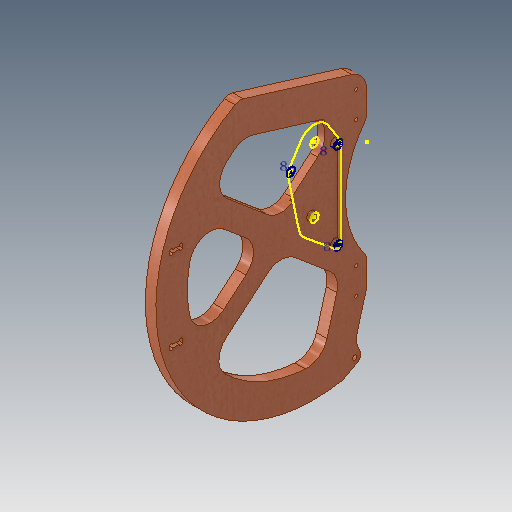
# Autodesk Inventor part: Tplate
Saved by Autodesk Inventor 2019.4 (Build 234330000, 330)
## iProperties
Created: 2019-06-12
Part Number: Tplate
Material: 木材(クルミ)
Document SubType Name: Modeling
Designer: AzLIer
Density: 0.55 g/cm^3
Appearance: クルミ材 - ナチュラル つや出し
Mass: 145.761 g
Surface Area: 731.193 cm^2
Volume: 265.02 cm^3
Author: AzLIer
Autodesk Inventor part; units mm, degrees
(part 1 of 3)
ref_plane "YZ Plane" through (0, 0, 0) normal (1, 0, 0) x (0, 1, 0)
ref_plane "XZ Plane" through (0, 0, 0) normal (0, 1, 0) x (-1, 0, 0)
ref_plane "XY Plane" through (0, 0, 0) normal (0, 0, 1) x (1, 0, 0)
sketch "スケッチ2" plane through (0, 0, 0) normal (1, 0, 0) x (0, 1, 0)
  line L0 (151.996, 0) -> (-248.004, 0)
  line L1 (-248.004, 0) -> (-248.004, 200)
  line L2 (-248.004, 200) -> (151.996, 200)
  line L3 (151.996, 200) -> (151.996, 0)
  point P0 (0, 0)
  dimension "d5" = 400
  dimension "d6" = 200
  constraints: 8 end point, 2 parallel, 1 horizontal, 1 perpendicular, 1 point on line
  measures "d5" distance of L1.end L2.end
  measures "d6" distance of L0.end L1.end
extrude "押し出し2" add sketch "スケッチ2" along normal blind 10
sketch "スケッチ3" plane through (10, 0, 0) normal (1, 0, 0) x (0, 0, -1)
  circle A0 centre (-50, 24.7653) radius 4 projected
  circle A1 centre (-50, -37.0469) radius 4 projected
  circle A2 centre (-72.5, 11.9531) radius 1.6 projected
  circle A3 centre (-27.5, -71.0469) radius 1.6 projected
  circle A4 centre (-27.5, 11.9531) radius 1.6 projected
  line L0 (-62.6183, 32.8757) -> (-75.0237, 13.5752) projected
  arc A5 (-75.0237, 13.5752) -> (-75.4366, 11.3394) centre (-72.5, 11.9531) ccw projected
  line L1 (-75.4366, 11.3394) -> (-64.6828, -40.1155) projected
  arc A6 (-64.6828, -40.1155) -> (-59.5184, -48.64) centre (-50, -37.0469) ccw projected
  line L2 (-59.5184, -48.64) -> (-29.4037, -73.3655) projected
  arc A7 (-29.4037, -73.3655) -> (-24.5, -71.0469) centre (-27.5, -71.0469) ccw projected
  line L3 (-24.5, -71.0469) -> (-24.5, 11.9531) projected
  arc A8 (-24.5, 11.9531) -> (-24.9763, 13.5752) centre (-27.5, 11.9531) ccw projected
  line L4 (-24.9763, 13.5752) -> (-37.3817, 32.8757) projected
  arc A9 (-37.3817, 32.8757) -> (-62.6183, 32.8757) centre (-50, 24.7653) ccw projected
  circle A10 centre (-27.5, -71.0469) radius 4
  circle A11 centre (-72.5, 11.9531) radius 4
  circle A12 centre (-27.5, 11.9531) radius 4
  point P0 (0, 0)
  dimension "d11" = 8
  dimension "d12" = 8
  dimension "d13" = 8
  constraints: 3 centre point, 3 coincident
  measures "d11" diameter of A10
  measures "d12" diameter of A11
  measures "d13" diameter of A12
extrude "押し出し3" cut sketch "スケッチ3" against normal blind 10 contours A0 | A1 | A2 | A3 | A4 | A11 L1 A5 L0 | L0 A5 L1 A11 | A12 L3 A8 L4 | L4 A8 L3 A12 | A10 L2 A7 L3 | L3 A7 L2 A10
extrude "押し出し4" cut sketch "スケッチ3" against normal blind 3 contours A9 L4 A12 L3 A10 L2 A6 L1 A11 L0 | A11 L1 A5 L0 | L4 A8 L3 A12 | L3 A7 L2 A10 picked at (-74.6765, 10.327) picked at (-25.0278, 10.8233) picked at (-25.0278, -69.9171)
sketch "スケッチ4" plane through (0, 0, 0) normal (-1, 0, 0) x (0, 0, 1)
  arc A0 (23.9528, -184.768) -> (125, 92.8569) centre (50, -37.0469) ccw projected
  circle A1 centre (50, -37.0469) radius 150
  point P0 (0, 0)
  constraints: 1 centre point, 1 coincident, 1 concentric
extrude "押し出し5" cut sketch "スケッチ4" against normal through all keep common part
sketch "スケッチ5" plane through (0, 0, 0) normal (-1, 0, 0) x (0, 0, 1)
  line L0 (0, 57.9531) -> (20, 57.9531) projected
  arc A0 (23.9528, -184.768) -> (125, 92.8569) centre (50, -37.0469) ccw projected
  arc A1 (27.4257, -165.0719) -> (23.9528, -184.768) centre (25.6893, -174.92) ccw projected
  arc A2 (27.4257, -165.0719) -> (115, 75.5364) centre (50, -37.0469) ccw projected
  arc A3 (125, 92.8569) -> (115, 75.5364) centre (120, 84.1967) ccw projected
  line L1 (0, 57.9531) -> (117.0753, 93.7594)
  line L2 (0, -120) -> (16.0565, -177.605)
  line L3 (0, 57.9531) -> (0, -120)
  point P0 (0, 0)
  dimension "d57" = 120
  constraints: 6 end point, 2 point on circle, 2 tangent, 1 vertical
  measures "d57" distance of point (0, 0) L2.start
extrude "押し出し6" cut sketch "スケッチ5" against normal through all keep common part
sketch "スケッチ6" plane through (0, 0, 0) normal (-1, 0, 0) x (0, 0, 1)
  circle A0 centre (10, -97.0469) radius 1.6 projected
  circle A1 centre (10, 47.9531) radius 1.6 projected
  circle A2 centre (10, 22.9531) radius 1.6 projected
  circle A3 centre (10, -122.0469) radius 1.6 projected
  point P0 (0, 0)
hole "穴1" at (0, 47.9531, 10) at (0, 22.9531, 10) at (0, -97.0469, 10) at (0, -122.0469, 10) direction (1, 0, 0) diameter 3.2 end through all
sketch "スケッチ7" plane through (0, 0, 0) normal (-1, 0, 0) x (0, 0, 1)
  circle A0 centre (186.0293, -60.2852) radius 1.6 construction
  circle A1 centre (83.5145, -42.7723) radius 1.6 construction
  circle A2 centre (98.3003, -45.2982) radius 1.6 construction
  circle A3 centre (171.2435, -57.7593) radius 1.6 construction
  line L0 (76.8917, -34.0322) -> (74.3658, -48.818) construction
  line L1 (76.8917, -34.0322) -> (195.1781, -54.2394) construction
  line L2 (192.6522, -69.0252) -> (195.1781, -54.2394) construction
  line L3 (74.3658, -48.818) -> (192.6522, -69.0252) construction
  circle A4 centre (191.638, 32.9722) radius 1.6 construction
  circle A5 centre (80.4791, -21.9795) radius 1.6 construction
  circle A6 centre (93.9257, -15.3321) radius 1.6 construction
  circle A7 centre (173.7092, 24.109) radius 1.6 construction
  line L4 (69.9838, -18.8014) -> (76.6312, -32.2481) construction
  line L5 (69.9838, -18.8014) -> (195.4859, 43.2408) construction
  line L6 (202.1333, 29.7941) -> (195.4859, 43.2408) construction
  line L7 (76.6312, -32.2481) -> (202.1333, 29.7941) construction
  arc A8 (125.4318, -57.5418) -> (127.7114, -56.0453) centre (125.7686, -55.5703) ccw construction
  line L8 (125.4318, -57.5418) -> (85.6625, -50.7479) construction
  arc A9 (85.6625, -50.7479) -> (85.2499, -50.7207) centre (85.3257, -52.7193) ccw construction
  line L9 (85.2499, -50.7207) -> (50.5685, -52.0361) construction
  line L10 (50.5685, -52.0361) -> (16.9095, -54.9491) construction
  arc A10 (16.9095, -54.9491) -> (16.1379, -55.1785) centre (17.0819, -56.9416) ccw construction
  line L11 (16.1379, -55.1785) -> (12.8384, -56.9452) construction
  line L12 (12.7127, -57.0062) -> (12.8384, -56.9452) construction
  line L13 (12.365, -57.1532) -> (12.7127, -57.0062) construction
  line L14 (12.0042, -57.2757) -> (12.365, -57.1532) construction
  line L15 (11.6348, -57.3815) -> (12.0042, -57.2757) construction
  line L16 (11.2582, -57.4735) -> (11.6348, -57.3815) construction
  line L17 (10.8753, -57.5532) -> (11.2582, -57.4735) construction
  line L18 (10.4869, -57.6217) -> (10.8753, -57.5532) construction
  line L19 (10.0935, -57.6796) -> (10.4869, -57.6217) construction
  line L20 (9.6953, -57.7276) -> (10.0935, -57.6796) construction
  line L21 (9.2927, -57.7659) -> (9.6953, -57.7276) construction
  line L22 (8.886, -57.7951) -> (9.2927, -57.7659) construction
  line L23 (8.4754, -57.8152) -> (8.886, -57.7951) construction
  line L24 (8.0611, -57.8266) -> (8.4754, -57.8152) construction
  line L25 (7.6433, -57.8294) -> (8.0611, -57.8266) construction
  line L26 (7.2222, -57.8238) -> (7.6433, -57.8294) construction
  line L27 (6.798, -57.8099) -> (7.2222, -57.8238) construction
  line L28 (6.3707, -57.7878) -> (6.798, -57.8099) construction
  line L29 (5.9406, -57.7577) -> (6.3707, -57.7878) construction
  line L30 (5.5078, -57.7195) -> (5.9406, -57.7577) construction
  line L31 (5.0724, -57.6734) -> (5.5078, -57.7195) construction
  line L32 (4.6346, -57.6194) -> (5.0724, -57.6734) construction
  line L33 (4.4858, -57.2882) -> (4.6346, -57.6194) construction
  line L34 (4.3395, -56.956) -> (4.4858, -57.2882) construction
  line L35 (4.1956, -56.6226) -> (4.3395, -56.956) construction
  line L36 (4.0542, -56.2883) -> (4.1956, -56.6226) construction
  line L37 (3.9151, -55.9529) -> (4.0542, -56.2883) construction
  line L38 (3.7786, -55.6165) -> (3.9151, -55.9529) construction
  line L39 (3.6445, -55.2791) -> (3.7786, -55.6165) construction
  line L40 (3.5128, -54.9408) -> (3.6445, -55.2791) construction
  line L41 (3.3836, -54.6015) -> (3.5128, -54.9408) construction
  line L42 (3.2569, -54.2613) -> (3.3836, -54.6015) construction
  line L43 (3.5307, -53.9154) -> (3.2569, -54.2613) construction
  line L44 (3.8083, -53.5767) -> (3.5307, -53.9154) construction
  line L45 (4.0896, -53.2456) -> (3.8083, -53.5767) construction
  line L46 (4.3746, -52.9221) -> (4.0896, -53.2456) construction
  line L47 (4.6632, -52.6063) -> (4.3746, -52.9221) construction
  line L48 (4.9555, -52.2985) -> (4.6632, -52.6063) construction
  line L49 (5.2513, -51.9988) -> (4.9555, -52.2985) construction
  line L50 (5.5507, -51.7074) -> (5.2513, -51.9988) construction
  line L51 (5.8536, -51.4245) -> (5.5507, -51.7074) construction
  line L52 (6.1601, -51.1505) -> (5.8536, -51.4245) construction
  line L53 (6.4701, -50.8856) -> (6.1601, -51.1505) construction
  line L54 (6.7836, -50.6302) -> (6.4701, -50.8856) construction
  line L55 (7.1007, -50.3847) -> (6.7836, -50.6302) construction
  line L56 (7.4216, -50.1496) -> (7.1007, -50.3847) construction
  line L57 (7.7461, -49.9256) -> (7.4216, -50.1496) construction
  line L58 (8.0746, -49.7135) -> (7.7461, -49.9256) construction
  line L59 (8.4073, -49.5144) -> (8.0746, -49.7135) construction
  line L60 (8.7447, -49.3303) -> (8.4073, -49.5144) construction
  line L61 (9.0875, -49.1641) -> (8.7447, -49.3303) construction
  line L62 (9.4383, -49.0246) -> (9.0875, -49.1641) construction
  line L63 (9.7029, -48.935) -> (9.4383, -49.0246) construction
  line L64 (9.956, -48.8366) -> (9.7029, -48.935) construction
  line L65 (10.1978, -48.7316) -> (9.956, -48.8366) construction
  line L66 (10.4291, -48.6228) -> (10.1978, -48.7316) construction
  line L67 (10.648, -48.5048) -> (10.4291, -48.6228) construction
  line L68 (10.8544, -48.3775) -> (10.648, -48.5048) construction
  line L69 (11.048, -48.2408) -> (10.8544, -48.3775) construction
  line L70 (11.2303, -48.1008) -> (11.048, -48.2408) construction
  line L71 (11.3993, -47.9514) -> (11.2303, -48.1008) construction
  line L72 (11.5542, -47.7908) -> (11.3993, -47.9514) construction
  line L73 (11.6966, -47.6261) -> (11.5542, -47.7908) construction
  line L74 (11.8245, -47.451) -> (11.6966, -47.6261) construction
  line L75 (11.9375, -47.2663) -> (11.8245, -47.451) construction
  line L76 (12.036, -47.0751) -> (11.9375, -47.2663) construction
  line L77 (12.1174, -46.8705) -> (12.036, -47.0751) construction
  line L78 (12.1829, -46.6599) -> (12.1174, -46.8705) construction
  line L79 (12.2282, -46.4321) -> (12.1829, -46.6599) construction
  line L80 (12.2532, -46.1928) -> (12.2282, -46.4321) construction
  line L81 (12.2494, -45.9198) -> (12.2532, -46.1928) construction
  line L82 (12.2003, -45.576) -> (12.2494, -45.9198) construction
  line L83 (12.1882, -45.5219) -> (12.2003, -45.576) construction
  line L84 (12.1761, -45.4679) -> (12.1882, -45.5219) construction
  line L85 (12.1641, -45.4138) -> (12.1761, -45.4679) construction
  line L86 (12.1521, -45.3596) -> (12.1641, -45.4138) construction
  line L87 (12.1403, -45.3055) -> (12.1521, -45.3596) construction
  line L88 (12.1285, -45.2513) -> (12.1403, -45.3055) construction
  line L89 (12.1168, -45.1972) -> (12.1285, -45.2513) construction
  line L90 (12.1052, -45.143) -> (12.1168, -45.1972) construction
  line L91 (12.0937, -45.0888) -> (12.1052, -45.143) construction
  line L92 (12.0822, -45.0346) -> (12.0937, -45.0888) construction
  line L93 (11.9836, -44.7016) -> (12.0822, -45.0346) construction
  line L94 (11.8734, -44.4517) -> (11.9836, -44.7016) construction
  line L95 (11.7511, -44.2447) -> (11.8734, -44.4517) construction
  line L96 (11.615, -44.0564) -> (11.7511, -44.2447) construction
  line L97 (11.4677, -43.8922) -> (11.615, -44.0564) construction
  line L98 (11.3085, -43.7401) -> (11.4677, -43.8922) construction
  line L99 (11.1393, -43.6073) -> (11.3085, -43.7401) construction
  line L100 (10.9596, -43.4864) -> (11.1393, -43.6073) construction
  line L101 (10.7705, -43.3805) -> (10.9596, -43.4864) construction
  line L102 (10.5724, -43.29) -> (10.7705, -43.3805) construction
  line L103 (10.3647, -43.2085) -> (10.5724, -43.29) construction
  line L104 (10.1489, -43.1431) -> (10.3647, -43.2085) construction
  line L105 (9.9248, -43.0917) -> (10.1489, -43.1431) construction
  line L106 (9.6919, -43.048) -> (9.9248, -43.0917) construction
  line L107 (9.4512, -43.0183) -> (9.6919, -43.048) construction
  line L108 (9.203, -43.0022) -> (9.4512, -43.0183) construction
  line L109 (8.9474, -42.9996) -> (9.203, -43.0022) construction
  line L110 (8.6838, -43.0048) -> (8.9474, -42.9996) construction
  line L111 (8.4128, -43.0208) -> (8.6838, -43.0048) construction
  line L112 (8.1349, -43.0495) -> (8.4128, -43.0208) construction
  line L113 (7.7579, -43.0687) -> (8.1349, -43.0495) construction
  line L114 (7.377, -43.0604) -> (7.7579, -43.0687) construction
  line L115 (6.9936, -43.0335) -> (7.377, -43.0604) construction
  line L116 (6.6083, -42.9912) -> (6.9936, -43.0335) construction
  line L117 (6.2213, -42.9351) -> (6.6083, -42.9912) construction
  line L118 (5.8329, -42.8666) -> (6.2213, -42.9351) construction
  line L119 (5.4433, -42.7865) -> (5.8329, -42.8666) construction
  line L120 (5.0527, -42.6954) -> (5.4433, -42.7865) construction
  line L121 (4.6613, -42.5937) -> (5.0527, -42.6954) construction
  line L122 (4.2692, -42.482) -> (4.6613, -42.5937) construction
  line L123 (3.8764, -42.3605) -> (4.2692, -42.482) construction
  line L124 (3.4832, -42.2295) -> (3.8764, -42.3605) construction
  line L125 (3.0897, -42.0892) -> (3.4832, -42.2295) construction
  line L126 (2.6959, -41.94) -> (3.0897, -42.0892) construction
  line L127 (2.302, -41.7818) -> (2.6959, -41.94) construction
  line L128 (1.9081, -41.6149) -> (2.302, -41.7818) construction
  line L129 (1.5142, -41.4395) -> (1.9081, -41.6149) construction
  line L130 (1.1206, -41.2556) -> (1.5142, -41.4395) construction
  line L131 (0.7272, -41.0633) -> (1.1206, -41.2556) construction
  line L132 (0.3342, -40.8628) -> (0.7272, -41.0633) construction
  line L133 (0.3077, -40.5008) -> (0.3342, -40.8628) construction
  line L134 (0.2839, -40.1385) -> (0.3077, -40.5008) construction
  line L135 (0.2626, -39.7761) -> (0.2839, -40.1385) construction
  line L136 (0.2441, -39.4135) -> (0.2626, -39.7761) construction
  line L137 (0.2282, -39.0508) -> (0.2441, -39.4135) construction
  line L138 (0.2149, -38.688) -> (0.2282, -39.0508) construction
  line L139 (0.2042, -38.3251) -> (0.2149, -38.688) construction
  line L140 (0.1962, -37.9621) -> (0.2042, -38.3251) construction
  line L141 (0.1909, -37.5991) -> (0.1962, -37.9621) construction
  line L142 (0.1882, -37.2361) -> (0.1909, -37.5991) construction
  line L143 (0.5638, -37.0046) -> (0.1882, -37.2361) construction
  line L144 (0.9404, -36.7814) -> (0.5638, -37.0046) construction
  line L145 (1.318, -36.5664) -> (0.9404, -36.7814) construction
  line L146 (1.6965, -36.3599) -> (1.318, -36.5664) construction
  line L147 (2.0757, -36.1619) -> (1.6965, -36.3599) construction
  line L148 (2.4556, -35.9726) -> (2.0757, -36.1619) construction
  line L149 (2.8361, -35.7921) -> (2.4556, -35.9726) construction
  line L150 (3.2171, -35.6207) -> (2.8361, -35.7921) construction
  line L151 (3.5985, -35.4585) -> (3.2171, -35.6207) construction
  line L152 (3.9802, -35.3058) -> (3.5985, -35.4585) construction
  line L153 (4.3621, -35.1629) -> (3.9802, -35.3058) construction
  line L154 (4.7441, -35.0301) -> (4.3621, -35.1629) construction
  line L155 (5.1261, -34.9079) -> (4.7441, -35.0301) construction
  line L156 (5.508, -34.7967) -> (5.1261, -34.9079) construction
  line L157 (5.8896, -34.6972) -> (5.508, -34.7967) construction
  line L158 (6.2708, -34.6102) -> (5.8896, -34.6972) construction
  line L159 (6.6515, -34.537) -> (6.2708, -34.6102) construction
  line L160 (7.0315, -34.4794) -> (6.6515, -34.537) construction
  line L161 (7.4105, -34.4405) -> (7.0315, -34.4794) construction
  line L162 (7.7879, -34.4294) -> (7.4105, -34.4405) construction
  line L163 (8.0672, -34.4356) -> (7.7879, -34.4294) construction
  line L164 (8.3386, -34.4298) -> (8.0672, -34.4356) construction
  line L165 (8.6017, -34.4138) -> (8.3386, -34.4298) construction
  line L166 (8.8563, -34.3906) -> (8.6017, -34.4138) construction
  line L167 (9.1024, -34.3546) -> (8.8563, -34.3906) construction
  line L168 (9.3399, -34.3056) -> (9.1024, -34.3546) construction
  line L169 (9.5686, -34.2434) -> (9.3399, -34.3056) construction
  line L170 (9.7878, -34.1741) -> (9.5686, -34.2434) construction
  line L171 (9.9976, -34.0916) -> (9.7878, -34.1741) construction
  line L172 (10.1981, -33.9937) -> (9.9976, -34.0916) construction
  line L173 (10.3883, -33.8876) -> (10.1981, -33.9937) construction
  line L174 (10.5683, -33.7668) -> (10.3883, -33.8876) construction
  line L175 (10.7377, -33.6318) -> (10.5683, -33.7668) construction
  line L176 (10.8956, -33.4859) -> (10.7377, -33.6318) construction
  line L177 (11.0421, -33.3215) -> (10.8956, -33.4859) construction
  line L178 (11.1757, -33.1459) -> (11.0421, -33.3215) construction
  line L179 (11.2962, -32.9474) -> (11.1757, -33.1459) construction
  line L180 (11.4015, -32.7311) -> (11.2962, -32.9474) construction
  line L181 (11.4913, -32.4732) -> (11.4015, -32.7311) construction
  line L182 (11.5628, -32.1334) -> (11.4913, -32.4732) construction
  line L183 (11.5698, -32.0784) -> (11.5628, -32.1334) construction
  line L184 (11.577, -32.0235) -> (11.5698, -32.0784) construction
  line L185 (11.5842, -31.9685) -> (11.577, -32.0235) construction
  line L186 (11.5915, -31.9136) -> (11.5842, -31.9685) construction
  line L187 (11.5989, -31.8587) -> (11.5915, -31.9136) construction
  line L188 (11.6064, -31.8037) -> (11.5989, -31.8587) construction
  line L189 (11.6139, -31.7488) -> (11.6064, -31.8037) construction
  line L190 (11.6215, -31.6939) -> (11.6139, -31.7488) construction
  line L191 (11.6292, -31.6391) -> (11.6215, -31.6939) construction
  line L192 (11.637, -31.5842) -> (11.6292, -31.6391) construction
  line L193 (11.6582, -31.2376) -> (11.637, -31.5842) construction
  line L194 (11.6401, -30.9651) -> (11.6582, -31.2376) construction
  line L195 (11.596, -30.7287) -> (11.6401, -30.9651) construction
  line L196 (11.5325, -30.5052) -> (11.596, -30.7287) construction
  line L197 (11.4503, -30.3005) -> (11.5325, -30.5052) construction
  line L198 (11.3527, -30.1032) -> (11.4503, -30.3005) construction
  line L199 (11.2391, -29.9206) -> (11.3527, -30.1032) construction
  line L200 (11.1116, -29.7455) -> (11.2391, -29.9206) construction
  line L201 (10.9701, -29.5812) -> (11.1116, -29.7455) construction
  line L202 (10.8149, -29.4285) -> (10.9701, -29.5812) construction
  line L203 (10.6476, -29.2809) -> (10.8149, -29.4285) construction
  line L204 (10.4671, -29.1456) -> (10.6476, -29.2809) construction
  line L205 (10.2742, -29.0206) -> (10.4671, -29.1456) construction
  line L206 (10.0702, -28.8999) -> (10.2742, -29.0206) construction
  line L207 (9.8543, -28.7897) -> (10.0702, -28.8999) construction
  line L208 (9.6265, -28.6896) -> (9.8543, -28.7897) construction
  line L209 (9.3872, -28.5998) -> (9.6265, -28.6896) construction
  line L210 (9.1378, -28.5145) -> (9.3872, -28.5998) construction
  line L211 (8.8777, -28.4369) -> (9.1378, -28.5145) construction
  line L212 (8.6067, -28.3688) -> (8.8777, -28.4369) construction
  line L213 (8.2458, -28.2579) -> (8.6067, -28.3688) construction
  line L214 (7.8907, -28.1199) -> (8.2458, -28.2579) construction
  line L215 (7.5397, -27.9634) -> (7.8907, -28.1199) construction
  line L216 (7.192, -27.7918) -> (7.5397, -27.9634) construction
  line L217 (6.8475, -27.6068) -> (7.192, -27.7918) construction
  line L218 (6.506, -27.4096) -> (6.8475, -27.6068) construction
  line L219 (6.1673, -27.2011) -> (6.506, -27.4096) construction
  line L220 (5.8315, -26.9818) -> (6.1673, -27.2011) construction
  line L221 (5.4984, -26.7524) -> (5.8315, -26.9818) construction
  line L222 (5.1681, -26.5133) -> (5.4984, -26.7524) construction
  line L223 (4.8407, -26.2648) -> (5.1681, -26.5133) construction
  line L224 (4.516, -26.0073) -> (4.8407, -26.2648) construction
  line L225 (4.1941, -25.7409) -> (4.516, -26.0073) construction
  line L226 (3.8752, -25.4659) -> (4.1941, -25.7409) construction
  line L227 (3.5591, -25.1826) -> (3.8752, -25.4659) construction
  line L228 (3.246, -24.891) -> (3.5591, -25.1826) construction
  line L229 (2.9359, -24.5915) -> (3.246, -24.891) construction
  line L230 (2.6289, -24.284) -> (2.9359, -24.5915) construction
  line L231 (2.325, -23.9688) -> (2.6289, -24.284) construction
  line L232 (2.0243, -23.646) -> (2.325, -23.9688) construction
  line L233 (2.1232, -23.2967) -> (2.0243, -23.646) construction
  line L234 (2.2247, -22.9481) -> (2.1232, -23.2967) construction
  line L235 (2.3287, -22.6003) -> (2.2247, -22.9481) construction
  line L236 (2.4353, -22.2532) -> (2.3287, -22.6003) construction
  line L237 (2.5444, -21.907) -> (2.4353, -22.2532) construction
  line L238 (2.656, -21.5615) -> (2.5444, -21.907) construction
  line L239 (2.7701, -21.2168) -> (2.656, -21.5615) construction
  line L240 (2.8867, -20.873) -> (2.7701, -21.2168) construction
  line L241 (3.0059, -20.5301) -> (2.8867, -20.873) construction
  line L242 (3.1275, -20.188) -> (3.0059, -20.5301) construction
  line L243 (3.5596, -20.099) -> (3.1275, -20.188) construction
  line L244 (3.9899, -20.018) -> (3.5596, -20.099) construction
  line L245 (4.4183, -19.9452) -> (3.9899, -20.018) construction
  line L246 (4.8445, -19.8805) -> (4.4183, -19.9452) construction
  line L247 (5.2686, -19.8242) -> (4.8445, -19.8805) construction
  line L248 (5.6904, -19.7762) -> (5.2686, -19.8242) construction
  line L249 (6.1096, -19.7368) -> (5.6904, -19.7762) construction
  line L250 (6.5263, -19.706) -> (6.1096, -19.7368) construction
  line L251 (6.9401, -19.6841) -> (6.5263, -19.706) construction
  line L252 (7.351, -19.6711) -> (6.9401, -19.6841) construction
  line L253 (7.7588, -19.6675) -> (7.351, -19.6711) construction
  line L254 (8.1631, -19.6733) -> (7.7588, -19.6675) construction
  line L255 (8.5639, -19.6891) -> (8.1631, -19.6733) construction
  line L256 (8.9608, -19.7152) -> (8.5639, -19.6891) construction
  line L257 (9.3534, -19.7522) -> (8.9608, -19.7152) construction
  line L258 (9.7414, -19.8009) -> (9.3534, -19.7522) construction
  line L259 (10.1242, -19.8624) -> (9.7414, -19.8009) construction
  line L260 (10.501, -19.9381) -> (10.1242, -19.8624) construction
  line L261 (10.8704, -20.0312) -> (10.501, -19.9381) construction
  line L262 (11.2288, -20.1498) -> (10.8704, -20.0312) construction
  line L263 (11.4891, -20.2512) -> (11.2288, -20.1498) construction
  line L264 (11.7462, -20.3386) -> (11.4891, -20.2512) construction
  line L265 (11.9989, -20.4135) -> (11.7462, -20.3386) construction
  line L266 (12.246, -20.4789) -> (11.9989, -20.4135) construction
  line L267 (12.4896, -20.5292) -> (12.246, -20.4789) construction
  line L268 (12.7295, -20.5644) -> (12.4896, -20.5292) construction
  line L269 (12.9657, -20.5841) -> (12.7295, -20.5644) construction
  line L270 (13.1954, -20.594) -> (12.9657, -20.5841) construction
  line L271 (13.4209, -20.5882) -> (13.1954, -20.594) construction
  line L272 (13.6427, -20.5647) -> (13.4209, -20.5882) construction
  line L273 (13.8577, -20.5301) -> (13.6427, -20.5647) construction
  line L274 (14.0682, -20.4781) -> (13.8577, -20.5301) construction
  line L275 (14.2735, -20.4093) -> (14.0682, -20.4781) construction
  line L276 (14.4719, -20.3261) -> (14.2735, -20.4093) construction
  line L277 (14.6658, -20.2218) -> (14.4719, -20.3261) construction
  line L278 (14.8513, -20.1025) -> (14.6658, -20.2218) construction
  line L279 (15.0325, -19.9571) -> (14.8513, -20.1025) construction
  line L280 (15.2054, -19.7899) -> (15.0325, -19.9571) construction
  line L281 (15.3779, -19.5783) -> (15.2054, -19.7899) construction
  line L282 (15.5613, -19.2834) -> (15.3779, -19.5783) construction
  line L283 (15.5868, -19.2342) -> (15.5613, -19.2834) construction
  line L284 (15.6123, -19.185) -> (15.5868, -19.2342) construction
  line L285 (15.6379, -19.1358) -> (15.6123, -19.185) construction
  line L286 (15.6635, -19.0867) -> (15.6379, -19.1358) construction
  line L287 (15.6892, -19.0376) -> (15.6635, -19.0867) construction
  line L288 (15.715, -18.9885) -> (15.6892, -19.0376) construction
  line L289 (15.7409, -18.9395) -> (15.715, -18.9885) construction
  line L290 (15.7668, -18.8906) -> (15.7409, -18.9395) construction
  line L291 (15.7928, -18.8416) -> (15.7668, -18.8906) construction
  line L292 (15.8189, -18.7927) -> (15.7928, -18.8416) construction
  line L293 (15.9574, -18.4743) -> (15.8189, -18.7927) construction
  line L294 (16.0336, -18.212) -> (15.9574, -18.4743) construction
  line L295 (16.073, -17.9748) -> (16.0336, -18.212) construction
  line L296 (16.0897, -17.7431) -> (16.073, -17.9748) construction
  line L297 (16.0825, -17.5226) -> (16.0897, -17.7431) construction
  line L298 (16.0583, -17.3038) -> (16.0825, -17.5226) construction
  line L299 (16.014, -17.0933) -> (16.0583, -17.3038) construction
  line L300 (15.9541, -16.8852) -> (16.014, -17.0933) construction
  line L301 (15.8773, -16.6824) -> (15.9541, -16.8852) construction
  line L302 (15.7837, -16.4858) -> (15.8773, -16.6824) construction
  line L303 (15.677, -16.2899) -> (15.7837, -16.4858) construction
  line L304 (15.5537, -16.101) -> (15.677, -16.2899) construction
  line L305 (15.4151, -15.9177) -> (15.5537, -16.101) construction
  line L306 (15.2647, -15.7345) -> (15.4151, -15.9177) construction
  line L307 (15.0995, -15.557) -> (15.2647, -15.7345) construction
  line L308 (14.9197, -15.3851) -> (15.0995, -15.557) construction
  line L309 (14.7256, -15.2188) -> (14.9197, -15.3851) construction
  line L310 (14.5203, -15.0534) -> (14.7256, -15.2188) construction
  line L311 (14.3024, -14.8914) -> (14.5203, -15.0534) construction
  line L312 (14.0711, -14.7348) -> (14.3024, -14.8914) construction
  line L313 (13.7699, -14.5072) -> (14.0711, -14.7348) construction
  line L314 (13.4835, -14.256) -> (13.7699, -14.5072) construction
  line L315 (13.2071, -13.9889) -> (13.4835, -14.256) construction
  line L316 (12.9391, -13.7088) -> (13.2071, -13.9889) construction
  line L317 (12.6786, -13.4171) -> (12.9391, -13.7088) construction
  line L318 (12.4252, -13.115) -> (12.6786, -13.4171) construction
  line L319 (12.1782, -12.8032) -> (12.4252, -13.115) construction
  line L320 (11.9376, -12.4823) -> (12.1782, -12.8032) construction
  line L321 (11.7031, -12.1528) -> (11.9376, -12.4823) construction
  line L322 (11.4745, -11.8152) -> (11.7031, -12.1528) construction
  line L323 (11.2518, -11.4697) -> (11.4745, -11.8152) construction
  line L324 (11.0348, -11.1166) -> (11.2518, -11.4697) construction
  line L325 (10.8234, -10.7562) -> (11.0348, -11.1166) construction
  line L326 (10.6178, -10.3887) -> (10.8234, -10.7562) construction
  line L327 (10.4177, -10.0144) -> (10.6178, -10.3887) construction
  line L328 (10.2232, -9.6333) -> (10.4177, -10.0144) construction
  line L329 (10.0342, -9.2458) -> (10.2232, -9.6333) construction
  line L330 (9.8509, -8.8518) -> (10.0342, -9.2458) construction
  line L331 (9.6731, -8.4517) -> (9.8509, -8.8518) construction
  line L332 (9.5009, -8.0455) -> (9.6731, -8.4517) construction
  line L333 (9.7134, -7.7511) -> (9.5009, -8.0455) construction
  line L334 (9.928, -7.4583) -> (9.7134, -7.7511) construction
  line L335 (10.1447, -7.167) -> (9.928, -7.4583) construction
  line L336 (10.3635, -6.8773) -> (10.1447, -7.167) construction
  line L337 (10.5845, -6.5892) -> (10.3635, -6.8773) construction
  line L338 (10.8075, -6.3028) -> (10.5845, -6.5892) construction
  line L339 (11.0326, -6.0179) -> (10.8075, -6.3028) construction
  line L340 (11.2598, -5.7347) -> (11.0326, -6.0179) construction
  line L341 (11.4891, -5.4532) -> (11.2598, -5.7347) construction
  line L342 (11.7203, -5.1734) -> (11.4891, -5.4532) construction
  line L343 (12.1568, -5.2375) -> (11.7203, -5.1734) construction
  line L344 (12.5889, -5.3086) -> (12.1568, -5.2375) construction
  line L345 (13.0163, -5.3867) -> (12.5889, -5.3086) construction
  line L346 (13.439, -5.4717) -> (13.0163, -5.3867) construction
  line L347 (13.8568, -5.5638) -> (13.439, -5.4717) construction
  line L348 (14.2695, -5.663) -> (13.8568, -5.5638) construction
  line L349 (14.677, -5.7693) -> (14.2695, -5.663) construction
  line L350 (15.079, -5.8829) -> (14.677, -5.7693) construction
  line L351 (15.4754, -6.0038) -> (15.079, -5.8829) construction
  line L352 (15.8659, -6.1322) -> (15.4754, -6.0038) construction
  line L353 (16.2503, -6.2682) -> (15.8659, -6.1322) construction
  line L354 (16.6283, -6.412) -> (16.2503, -6.2682) construction
  line L355 (16.9995, -6.5639) -> (16.6283, -6.412) construction
  line L356 (17.3635, -6.7242) -> (16.9995, -6.5639) construction
  line L357 (17.7198, -6.8933) -> (17.3635, -6.7242) construction
  line L358 (18.0677, -7.0717) -> (17.7198, -6.8933) construction
  line L359 (18.4064, -7.2604) -> (18.0677, -7.0717) construction
  line L360 (18.7346, -7.4605) -> (18.4064, -7.2604) construction
  line L361 (19.0499, -7.6743) -> (18.7346, -7.4605) construction
  line L362 (19.3461, -7.9083) -> (19.0499, -7.6743) construction
  line L363 (19.5561, -8.0926) -> (19.3461, -7.9083) construction
  line L364 (19.7677, -8.2626) -> (19.5561, -8.0926) construction
  line L365 (19.9796, -8.4195) -> (19.7677, -8.2626) construction
  line L366 (20.1895, -8.5654) -> (19.9796, -8.4195) construction
  line L367 (20.4012, -8.696) -> (20.1895, -8.5654) construction
  line L368 (20.6146, -8.8111) -> (20.4012, -8.696) construction
  line L369 (20.8298, -8.9104) -> (20.6146, -8.8111) construction
  line L370 (21.0422, -8.9983) -> (20.8298, -8.9104) construction
  line L371 (21.256, -9.07) -> (21.0422, -8.9983) construction
  line L372 (21.4726, -9.1238) -> (21.256, -9.07) construction
  line L373 (21.6864, -9.1648) -> (21.4726, -9.1238) construction
  line L374 (21.902, -9.188) -> (21.6864, -9.1648) construction
  line L375 (22.1185, -9.1935) -> (21.902, -9.188) construction
  line L376 (22.3333, -9.1832) -> (22.1185, -9.1935) construction
  line L377 (22.5512, -9.1514) -> (22.3333, -9.1832) construction
  line L378 (22.7663, -9.1028) -> (22.5512, -9.1514) construction
  line L379 (22.9863, -9.0282) -> (22.7663, -9.1028) construction
  line L380 (23.206, -8.9302) -> (22.9863, -9.0282) construction
  line L381 (23.4405, -8.7903) -> (23.206, -8.9302) construction
  line L382 (23.7137, -8.576) -> (23.4405, -8.7903) construction
  line L383 (23.7545, -8.5384) -> (23.7137, -8.576) construction
  line L384 (23.7953, -8.5009) -> (23.7545, -8.5384) construction
  line L385 (23.8361, -8.4634) -> (23.7953, -8.5009) construction
  line L386 (23.877, -8.426) -> (23.8361, -8.4634) construction
  line L387 (23.918, -8.3887) -> (23.877, -8.426) construction
  line L388 (23.959, -8.3514) -> (23.918, -8.3887) construction
  line L389 (24.0001, -8.3142) -> (23.959, -8.3514) construction
  line L390 (24.0412, -8.2771) -> (24.0001, -8.3142) construction
  line L391 (24.0823, -8.24) -> (24.0412, -8.2771) construction
  line L392 (24.1236, -8.2029) -> (24.0823, -8.24) construction
  line L393 (24.3626, -7.9511) -> (24.1236, -8.2029) construction
  line L394 (24.5239, -7.7307) -> (24.3626, -7.9511) construction
  line L395 (24.6421, -7.5212) -> (24.5239, -7.7307) construction
  line L396 (24.737, -7.3092) -> (24.6421, -7.5212) construction
  line L397 (24.8057, -7.0996) -> (24.737, -7.3092) construction
  line L398 (24.8578, -6.8857) -> (24.8057, -7.0996) construction
  line L399 (24.8881, -6.6728) -> (24.8578, -6.8857) construction
  line L400 (24.903, -6.4567) -> (24.8881, -6.6728) construction
  line L401 (24.9002, -6.2399) -> (24.903, -6.4567) construction
  line L402 (24.8795, -6.0231) -> (24.9002, -6.2399) construction
  line L403 (24.8462, -5.8025) -> (24.8795, -6.0231) construction
  line L404 (24.7949, -5.5829) -> (24.8462, -5.8025) construction
  line L405 (24.7274, -5.3632) -> (24.7949, -5.5829) construction
  line L406 (24.6488, -5.1396) -> (24.7274, -5.3632) construction
  line L407 (24.5542, -4.9163) -> (24.6488, -5.1396) construction
  line L408 (24.444, -4.6933) -> (24.5542, -4.9163) construction
  line L409 (24.3185, -4.4706) -> (24.444, -4.6933) construction
  line L410 (24.1822, -4.245) -> (24.3185, -4.4706) construction
  line L411 (24.0329, -4.0183) -> (24.1822, -4.245) construction
  line L412 (23.8691, -3.7919) -> (24.0329, -4.0183) construction
  line L413 (23.6639, -3.4751) -> (23.8691, -3.7919) construction
  line L414 (23.4806, -3.1411) -> (23.6639, -3.4751) construction
  line L415 (23.3122, -2.7956) -> (23.4806, -3.1411) construction
  line L416 (23.1562, -2.4407) -> (23.3122, -2.7956) construction
  line L417 (23.0113, -2.0775) -> (23.1562, -2.4407) construction
  line L418 (22.8764, -1.7069) -> (23.0113, -2.0775) construction
  line L419 (22.751, -1.3295) -> (22.8764, -1.7069) construction
  line L420 (22.6346, -0.9456) -> (22.751, -1.3295) construction
  line L421 (22.527, -0.5558) -> (22.6346, -0.9456) construction
  line L422 (22.4276, -0.1604) -> (22.527, -0.5558) construction
  line L423 (22.3365, 0.2405) -> (22.4276, -0.1604) construction
  line L424 (22.2533, 0.6465) -> (22.3365, 0.2405) construction
  line L425 (22.178, 1.0575) -> (22.2533, 0.6465) construction
  line L426 (22.1104, 1.4731) -> (22.178, 1.0575) construction
  line L427 (22.0504, 1.8933) -> (22.1104, 1.4731) construction
  line L428 (21.998, 2.3179) -> (22.0504, 1.8933) construction
  line L429 (21.953, 2.7467) -> (21.998, 2.3179) construction
  line L430 (21.9155, 3.1796) -> (21.953, 2.7467) construction
  line L431 (21.8853, 3.6164) -> (21.9155, 3.1796) construction
  line L432 (21.8624, 4.057) -> (21.8853, 3.6164) construction
  line L433 (22.1627, 4.261) -> (21.8624, 4.057) construction
  line L434 (22.4645, 4.4628) -> (22.1627, 4.261) construction
  line L435 (22.7678, 4.6623) -> (22.4645, 4.4628) construction
  line L436 (23.0725, 4.8597) -> (22.7678, 4.6623) construction
  line L437 (23.3786, 5.0549) -> (23.0725, 4.8597) construction
  line L438 (23.6862, 5.2478) -> (23.3786, 5.0549) construction
  line L439 (23.9952, 5.4384) -> (23.6862, 5.2478) construction
  line L440 (24.3055, 5.6268) -> (23.9952, 5.4384) construction
  line L441 (24.6172, 5.813) -> (24.3055, 5.6268) construction
  line L442 (24.9303, 5.9968) -> (24.6172, 5.813) construction
  line L443 (25.3185, 5.7873) -> (24.9303, 5.9968) construction
  line L444 (25.7002, 5.5727) -> (25.3185, 5.7873) construction
  line L445 (26.0751, 5.3532) -> (25.7002, 5.5727) construction
  line L446 (26.4432, 5.1287) -> (26.0751, 5.3532) construction
  line L447 (26.8043, 4.8992) -> (26.4432, 5.1287) construction
  line L448 (27.1582, 4.6649) -> (26.8043, 4.8992) construction
  line L449 (27.5047, 4.4256) -> (27.1582, 4.6649) construction
  line L450 (27.8437, 4.1814) -> (27.5047, 4.4256) construction
  line L451 (28.1748, 3.9322) -> (27.8437, 4.1814) construction
  line L452 (28.4979, 3.6779) -> (28.1748, 3.9322) construction
  line L453 (28.8126, 3.4187) -> (28.4979, 3.6779) construction
  line L454 (29.1186, 3.1542) -> (28.8126, 3.4187) construction
  line L455 (29.4155, 2.8845) -> (29.1186, 3.1542) construction
  line L456 (29.7027, 2.6094) -> (29.4155, 2.8845) construction
  line L457 (29.9797, 2.3287) -> (29.7027, 2.6094) construction
  line L458 (30.2456, 2.042) -> (29.9797, 2.3287) construction
  line L459 (30.4994, 1.7489) -> (30.2456, 2.042) construction
  line L460 (30.7393, 1.4487) -> (30.4994, 1.7489) construction
  line L461 (30.9624, 1.1399) -> (30.7393, 1.4487) construction
  line L462 (31.1607, 0.8187) -> (30.9624, 1.1399) construction
  line L463 (31.295, 0.5736) -> (31.1607, 0.8187) construction
  line L464 (31.4358, 0.3415) -> (31.295, 0.5736) construction
  line L465 (31.5812, 0.1216) -> (31.4358, 0.3415) construction
  line L466 (31.7285, -0.0873) -> (31.5812, 0.1216) construction
  line L467 (31.8828, -0.2824) -> (31.7285, -0.0873) construction
  line L468 (32.0439, -0.4636) -> (31.8828, -0.2824) construction
  line L469 (32.2122, -0.6305) -> (32.0439, -0.4636) construction
  line L470 (32.3817, -0.7857) -> (32.2122, -0.6305) construction
  line L471 (32.5582, -0.9262) -> (32.3817, -0.7857) construction
  line L472 (32.7432, -1.0508) -> (32.5582, -0.9262) construction
  line L473 (32.9302, -1.1625) -> (32.7432, -1.0508) construction
  line L474 (33.1248, -1.258) -> (32.9302, -1.1625) construction
  line L475 (33.3264, -1.3372) -> (33.1248, -1.258) construction
  line L476 (33.5318, -1.401) -> (33.3264, -1.3372) construction
  line L477 (33.7474, -1.4457) -> (33.5318, -1.401) construction
  line L478 (33.9662, -1.4736) -> (33.7474, -1.4457) construction
  line L479 (34.1984, -1.4787) -> (33.9662, -1.4736) construction
  line L480 (34.4383, -1.4617) -> (34.1984, -1.4787) construction
  line L481 (34.7066, -1.4105) -> (34.4383, -1.4617) construction
  line L482 (35.0366, -1.3025) -> (34.7066, -1.4105) construction
  line L483 (35.0877, -1.2812) -> (35.0366, -1.3025) construction
  line L484 (35.1389, -1.2599) -> (35.0877, -1.2812) construction
  line L485 (35.1901, -1.2387) -> (35.1389, -1.2599) construction
  line L486 (35.2413, -1.2175) -> (35.1901, -1.2387) construction
  line L487 (35.2926, -1.1964) -> (35.2413, -1.2175) construction
  line L488 (35.3439, -1.1754) -> (35.2926, -1.1964) construction
  line L489 (35.3952, -1.1545) -> (35.3439, -1.1754) construction
  line L490 (35.4465, -1.1337) -> (35.3952, -1.1545) construction
  line L491 (35.4979, -1.1129) -> (35.4465, -1.1337) construction
  line L492 (35.5493, -1.0922) -> (35.4979, -1.1129) construction
  line L493 (35.8601, -0.9373) -> (35.5493, -1.0922) construction
  line L494 (36.087, -0.7854) -> (35.8601, -0.9373) construction
  line L495 (36.2697, -0.6289) -> (36.087, -0.7854) construction
  line L496 (36.4315, -0.4622) -> (36.2697, -0.6289) construction
  line L497 (36.5677, -0.2887) -> (36.4315, -0.4622) construction
  line L498 (36.6898, -0.1054) -> (36.5677, -0.2887) construction
  line L499 (36.7911, 0.0842) -> (36.6898, -0.1054) construction
  line L500 (36.879, 0.2822) -> (36.7911, 0.0842) construction
  line L501 (36.9505, 0.4868) -> (36.879, 0.2822) construction
  line L502 (37.0052, 0.6976) -> (36.9505, 0.4868) construction
  line L503 (37.0494, 0.9163) -> (37.0052, 0.6976) construction
  line L504 (37.0763, 1.1402) -> (37.0494, 0.9163) construction
  line L505 (37.088, 1.3698) -> (37.0763, 1.1402) construction
  line L506 (37.0906, 1.6068) -> (37.088, 1.3698) construction
  line L507 (37.0781, 1.849) -> (37.0906, 1.6068) construction
  line L508 (37.0508, 2.0962) -> (37.0781, 1.849) construction
  line L509 (37.009, 2.3484) -> (37.0508, 2.0962) construction
  line L510 (36.9581, 2.607) -> (37.009, 2.3484) construction
  line L511 (36.8953, 2.8711) -> (36.9581, 2.607) construction
  line L512 (36.8188, 3.1398) -> (36.8953, 2.8711) construction
  line L513 (36.7344, 3.5078) -> (36.8188, 3.1398) construction
  line L514 (36.6764, 3.8843) -> (36.7344, 3.5078) construction
  line L515 (36.6363, 4.2666) -> (36.6764, 3.8843) construction
  line L516 (36.6111, 4.6534) -> (36.6363, 4.2666) construction
  line L517 (36.5991, 5.0443) -> (36.6111, 4.6534) construction
  line L518 (36.5991, 5.4387) -> (36.5991, 5.0443) construction
  line L519 (36.6104, 5.8362) -> (36.5991, 5.4387) construction
  line L520 (36.6323, 6.2367) -> (36.6104, 5.8362) construction
  line L521 (36.6645, 6.6398) -> (36.6323, 6.2367) construction
  line L522 (36.7064, 7.0454) -> (36.6645, 6.6398) construction
  line L523 (36.7579, 7.4533) -> (36.7064, 7.0454) construction
  line L524 (36.8186, 7.8632) -> (36.7579, 7.4533) construction
  line L525 (36.8884, 8.2752) -> (36.8186, 7.8632) construction
  line L526 (36.967, 8.6889) -> (36.8884, 8.2752) construction
  line L527 (37.0543, 9.1043) -> (36.967, 8.6889) construction
  line L528 (37.1503, 9.5212) -> (37.0543, 9.1043) construction
  line L529 (37.2547, 9.9395) -> (37.1503, 9.5212) construction
  line L530 (37.3674, 10.3591) -> (37.2547, 9.9395) construction
  line L531 (37.4884, 10.7799) -> (37.3674, 10.3591) construction
  line L532 (37.6176, 11.2017) -> (37.4884, 10.7799) construction
  line L533 (37.9696, 11.2907) -> (37.6176, 11.2017) construction
  line L534 (38.3222, 11.3771) -> (37.9696, 11.2907) construction
  line L535 (38.6755, 11.4609) -> (38.3222, 11.3771) construction
  line L536 (39.0293, 11.5422) -> (38.6755, 11.4609) construction
  line L537 (39.3838, 11.6208) -> (39.0293, 11.5422) construction
  line L538 (39.7387, 11.6969) -> (39.3838, 11.6208) construction
  line L539 (40.0943, 11.7704) -> (39.7387, 11.6969) construction
  line L540 (40.4503, 11.8413) -> (40.0943, 11.7704) construction
  line L541 (40.8069, 11.9096) -> (40.4503, 11.8413) construction
  line L542 (41.164, 11.9753) -> (40.8069, 11.9096) construction
  line L543 (41.4571, 11.6456) -> (41.164, 11.9753) construction
  line L544 (41.7424, 11.3135) -> (41.4571, 11.6456) construction
  line L545 (42.0196, 10.9789) -> (41.7424, 11.3135) construction
  line L546 (42.2888, 10.6421) -> (42.0196, 10.9789) construction
  line L547 (42.5496, 10.303) -> (42.2888, 10.6421) construction
  line L548 (42.802, 9.9617) -> (42.5496, 10.303) construction
  line L549 (43.0458, 9.6183) -> (42.802, 9.9617) construction
  line L550 (43.2808, 9.2729) -> (43.0458, 9.6183) construction
  line L551 (43.5067, 8.9255) -> (43.2808, 9.2729) construction
  line L552 (43.7234, 8.5761) -> (43.5067, 8.9255) construction
  line L553 (43.9304, 8.2248) -> (43.7234, 8.5761) construction
  line L554 (44.1275, 7.8717) -> (43.9304, 8.2248) construction
  line L555 (44.3142, 7.5167) -> (44.1275, 7.8717) construction
  line L556 (44.49, 7.16) -> (44.3142, 7.5167) construction
  line L557 (44.6543, 6.8014) -> (44.49, 7.16) construction
  line L558 (44.8061, 6.4411) -> (44.6543, 6.8014) construction
  line L559 (44.9443, 6.0789) -> (44.8061, 6.4411) construction
  line L560 (45.0671, 5.7146) -> (44.9443, 6.0789) construction
  line L561 (45.1712, 5.3482) -> (45.0671, 5.7146) construction
  line L562 (45.2477, 4.9785) -> (45.1712, 5.3482) construction
  line L563 (45.29, 4.7023) -> (45.2477, 4.9785) construction
  line L564 (45.3429, 4.4361) -> (45.29, 4.7023) construction
  line L565 (45.4044, 4.1797) -> (45.3429, 4.4361) construction
  line L566 (45.4714, 3.933) -> (45.4044, 4.1797) construction
  line L567 (45.5496, 3.6969) -> (45.4714, 3.933) construction
  line L568 (45.639, 3.4715) -> (45.5496, 3.6969) construction
  line L569 (45.7401, 3.2571) -> (45.639, 3.4715) construction
  line L570 (45.8463, 3.0533) -> (45.7401, 3.2571) construction
  line L571 (45.9641, 2.8609) -> (45.8463, 3.0533) construction
  line L572 (46.0953, 2.6805) -> (45.9641, 2.8609) construction
  line L573 (46.2328, 2.5116) -> (46.0953, 2.6805) construction
  line L574 (46.383, 2.3553) -> (46.2328, 2.5116) construction
  line L575 (46.5454, 2.212) -> (46.383, 2.3553) construction
  line L576 (46.7165, 2.0818) -> (46.5454, 2.212) construction
  line L577 (46.9038, 1.966) -> (46.7165, 2.0818) construction
  line L578 (47.0999, 1.865) -> (46.9038, 1.966) construction
  line L579 (47.3164, 1.7808) -> (47.0999, 1.865) construction
  line L580 (47.5477, 1.7146) -> (47.3164, 1.7808) construction
  line L581 (47.8172, 1.671) -> (47.5477, 1.7146) construction
  line L582 (48.1643, 1.6596) -> (47.8172, 1.671) construction
  line L583 (48.2197, 1.6622) -> (48.1643, 1.6596) construction
  line L584 (48.275, 1.6647) -> (48.2197, 1.6622) construction
  line L585 (48.3304, 1.6671) -> (48.275, 1.6647) construction
  line L586 (48.3858, 1.6695) -> (48.3304, 1.6671) construction
  line L587 (48.4411, 1.6717) -> (48.3858, 1.6695) construction
  line L588 (48.4965, 1.6739) -> (48.4411, 1.6717) construction
  line L589 (48.5519, 1.676) -> (48.4965, 1.6739) construction
  line L590 (48.6073, 1.6781) -> (48.5519, 1.676) construction
  line L591 (48.6626, 1.68) -> (48.6073, 1.6781) construction
  line L592 (48.718, 1.6819) -> (48.6626, 1.68) construction
  line L593 (49.0631, 1.7212) -> (48.718, 1.6819) construction
  line L594 (49.3283, 1.7863) -> (49.0631, 1.7212) construction
  line L595 (49.5534, 1.8708) -> (49.3283, 1.7863) construction
  line L596 (49.7624, 1.9722) -> (49.5534, 1.8708) construction
  line L597 (49.9498, 2.0887) -> (49.7624, 1.9722) construction
  line L598 (50.1272, 2.2191) -> (49.9498, 2.0887) construction
  line L599 (50.2873, 2.3626) -> (50.1272, 2.2191) construction
  line L600 (50.4376, 2.5186) -> (50.2873, 2.3626) construction
  line L601 (50.5748, 2.6865) -> (50.4376, 2.5186) construction
  line L602 (50.6983, 2.8658) -> (50.5748, 2.6865) construction
  line L603 (50.8146, 3.0562) -> (50.6983, 2.8658) construction
  line L604 (50.9165, 3.2574) -> (50.8146, 3.0562) construction
  line L605 (51.006, 3.4692) -> (50.9165, 3.2574) construction
  line L606 (51.0894, 3.691) -> (51.006, 3.4692) construction
  line L607 (51.1605, 3.9228) -> (51.0894, 3.691) construction
  line L608 (51.2195, 4.1645) -> (51.1605, 3.9228) construction
  line L609 (51.2664, 4.4157) -> (51.2195, 4.1645) construction
  line L610 (51.3071, 4.6762) -> (51.2664, 4.4157) construction
  line L611 (51.3384, 4.9458) -> (51.3071, 4.6762) construction
  line L612 (51.3584, 5.2245) -> (51.3384, 4.9458) construction
  line L613 (51.4049, 5.5992) -> (51.3584, 5.2245) construction
  line L614 (51.4792, 5.9728) -> (51.4049, 5.5992) construction
  line L615 (51.5723, 6.3457) -> (51.4792, 5.9728) construction
  line L616 (51.6809, 6.7179) -> (51.5723, 6.3457) construction
  line L617 (51.8033, 7.0893) -> (51.6809, 6.7179) construction
  line L618 (51.9382, 7.4598) -> (51.8033, 7.0893) construction
  line L619 (52.0848, 7.8296) -> (51.9382, 7.4598) construction
  line L620 (52.2424, 8.1984) -> (52.0848, 7.8296) construction
  line L621 (52.4104, 8.5662) -> (52.2424, 8.1984) construction
  line L622 (52.5886, 8.933) -> (52.4104, 8.5662) construction
  line L623 (52.7764, 9.2987) -> (52.5886, 8.933) construction
  line L624 (52.9737, 9.6631) -> (52.7764, 9.2987) construction
  line L625 (53.1801, 10.0264) -> (52.9737, 9.6631) construction
  line L626 (53.3955, 10.3882) -> (53.1801, 10.0264) construction
  line L627 (53.6197, 10.7487) -> (53.3955, 10.3882) construction
  line L628 (53.8524, 11.1076) -> (53.6197, 10.7487) construction
  line L629 (54.0936, 11.465) -> (53.8524, 11.1076) construction
  line L630 (54.3431, 11.8208) -> (54.0936, 11.465) construction
  line L631 (54.6007, 12.1748) -> (54.3431, 11.8208) construction
  line L632 (54.8664, 12.527) -> (54.6007, 12.1748) construction
  line L633 (55.2276, 12.4902) -> (54.8664, 12.527) construction
  line L634 (55.5885, 12.4508) -> (55.2276, 12.4902) construction
  line L635 (55.9491, 12.4088) -> (55.5885, 12.4508) construction
  line L636 (56.3094, 12.3641) -> (55.9491, 12.4088) construction
  line L637 (56.6693, 12.3168) -> (56.3094, 12.3641) construction
  line L638 (57.0289, 12.2669) -> (56.6693, 12.3168) construction
  line L639 (57.3882, 12.2143) -> (57.0289, 12.2669) construction
  line L640 (57.747, 12.1592) -> (57.3882, 12.2143) construction
  line L641 (58.1054, 12.1014) -> (57.747, 12.1592) construction
  line L642 (58.4634, 12.041) -> (58.1054, 12.1014) construction
  line L643 (58.6261, 11.6309) -> (58.4634, 12.041) construction
  line L644 (58.7806, 11.2212) -> (58.6261, 11.6309) construction
  line L645 (58.9267, 10.8121) -> (58.7806, 11.2212) construction
  line L646 (59.0644, 10.4035) -> (58.9267, 10.8121) construction
  line L647 (59.1935, 9.9956) -> (59.0644, 10.4035) construction
  line L648 (59.314, 9.5886) -> (59.1935, 9.9956) construction
  line L649 (59.4256, 9.1826) -> (59.314, 9.5886) construction
  line L650 (59.5283, 8.7776) -> (59.4256, 9.1826) construction
  line L651 (59.6218, 8.3738) -> (59.5283, 8.7776) construction
  line L652 (59.7059, 7.9714) -> (59.6218, 8.3738) construction
  line L653 (59.7803, 7.5705) -> (59.7059, 7.9714) construction
  line L654 (59.8447, 7.1713) -> (59.7803, 7.5705) construction
  line L655 (59.8988, 6.7739) -> (59.8447, 7.1713) construction
  line L656 (59.942, 6.3785) -> (59.8988, 6.7739) construction
  line L657 (59.9737, 5.9854) -> (59.942, 6.3785) construction
  line L658 (59.9931, 5.5948) -> (59.9737, 5.9854) construction
  line L659 (59.9991, 5.2072) -> (59.9931, 5.5948) construction
  line L660 (59.9899, 4.823) -> (59.9991, 5.2072) construction
  line L661 (59.9624, 4.443) -> (59.9899, 4.823) construction
  line L662 (59.9078, 4.0694) -> (59.9624, 4.443) construction
  line L663 (59.8531, 3.7954) -> (59.9078, 4.0694) construction
  line L664 (59.8118, 3.5272) -> (59.8531, 3.7954) construction
  line L665 (59.7818, 3.2652) -> (59.8118, 3.5272) construction
  line L666 (59.7604, 3.0105) -> (59.7818, 3.2652) construction
  line L667 (59.7531, 2.7619) -> (59.7604, 3.0105) construction
  line L668 (59.7602, 2.5195) -> (59.7531, 2.7619) construction
  line L669 (59.7818, 2.2835) -> (59.7602, 2.5195) construction
  line L670 (59.8119, 2.0556) -> (59.7818, 2.2835) construction
  line L671 (59.8567, 1.8346) -> (59.8119, 2.0556) construction
  line L672 (59.9184, 1.6201) -> (59.8567, 1.8346) construction
  line L673 (59.9898, 1.4144) -> (59.9184, 1.6201) construction
  line L674 (60.0775, 1.2162) -> (59.9898, 1.4144) construction
  line L675 (60.181, 1.0259) -> (60.0775, 1.2162) construction
  line L676 (60.2973, 0.845) -> (60.181, 1.0259) construction
  line L677 (60.4338, 0.6722) -> (60.2973, 0.845) construction
  line L678 (60.5835, 0.5102) -> (60.4338, 0.6722) construction
  line L679 (60.7581, 0.357) -> (60.5835, 0.5102) construction
  line L680 (60.9528, 0.2158) -> (60.7581, 0.357) construction
  line L681 (61.1912, 0.0826) -> (60.9528, 0.2158) construction
  line L682 (61.5134, -0.0468) -> (61.1912, 0.0826) construction
  line L683 (61.5663, -0.0633) -> (61.5134, -0.0468) construction